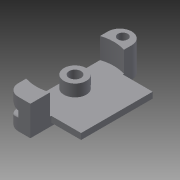
# Autodesk Inventor part: rodamiento
Saved by Autodesk Inventor 2015 SP1 (Build 190203100, 203)
## iProperties
Created: 2015-06-16
Part Number: rodamiento
Material: Generic
Document SubType Name: Modeling
Designer: pc
Density: 1 g/cm^3
Appearance: Default
Author: pc
Autodesk Inventor part; units mm, degrees
ref_plane "YZ Plane" through (0, 0, 0) normal (1, 0, 0) x (0, 1, 0)
ref_plane "XZ Plane" through (0, 0, 0) normal (0, 1, 0) x (-1, 0, 0)
ref_plane "XY Plane" through (0, 0, 0) normal (0, 0, 1) x (1, 0, 0)
sketch "Sketch1" plane through (0, 0, 0) normal (0, 0, 1) x (1, 0, 0)
  line L0 (0, -15) -> (0, 15) construction
  line L1 (-4, -15) -> (-4, 15)
  line L2 (4, 15) -> (4, -15)
  arc A0 (-4, -15) -> (0, -19) centre (0, -15) ccw
  arc A1 (4, 15) -> (-4, 15) centre (0, 15) ccw
  line L3 (4, -15) -> (0, -15)
  line L4 (-4, -11) -> (-4, -19)
  line L5 (-4, -19) -> (4, -19)
  line L6 (4, -19) -> (4, -15)
  point P0 (0, 0)
  point P1 (0, 0)
  dimension "d0" = 4
  dimension "d17" = 30
  constraints: 16 end point, 4 point on circle, 4 tangent, 3 parallel, 2 centre point, 2 midpoint, 1 coincident, 1 horizontal, 1 perpendicular, 1 point on line, 1 vertical
  measures "d0" radius of A0
  measures "d17" distance of L0.start L0.end
extrude "Extrusion1" add sketch "Sketch1" along normal blind 10 contours L1 A1 L2 L6 L5 A0
sketch "Sketch2" plane through (0, 0, 10) normal (0, 0, 1) x (1, 0, 0)
  line L0 (-4, 15) -> (-4, -15) projected
  arc A0 (-4, -15) -> (0, -19) centre (0, -15) ccw projected
  line L1 (4, -19) -> (4, 15) projected
  arc A1 (4, 15) -> (-4, 15) centre (0, 15) ccw projected
  circle A2 centre (0, 0) radius 13
  circle A3 centre (0, 0) radius 3.75
  line L2 (0, -19) -> (4, -19) projected
  dimension "d3" = 26
  dimension "d4" = 7.5
  constraints: 2 centre point, 2 coincident
  measures "d3" diameter of A2
  measures "d4" diameter of A3
extrude "Extrusion2" cut sketch "Sketch2" against normal blind 7 contours A2 L1 L0 | L0 A2 | A2 L1
sketch "Sketch3" plane through (0, 0, 10) normal (0, 0, 1) x (1, 0, 0)
  circle A0 centre (0, 0) radius 3.75 projected
  circle A1 centre (0, 0) radius 2
  line L0 (-4, 15) -> (-4, 12.3693) projected
  line L1 (4, -19) -> (4, -12.3693) projected
  arc A2 (4, 12.3693) -> (-4, 12.3693) centre (0, 0) ccw projected
  line L2 (4, 12.3693) -> (4, 15) projected
  arc A3 (4, 15) -> (-4, 15) centre (0, 15) ccw projected
  arc A4 (-4, -12.3693) -> (4, -12.3693) centre (0, 0) ccw projected
  line L3 (-4, -12.3693) -> (-4, -15) projected
  arc A5 (-4, -15) -> (0, -19) centre (0, -15) ccw projected
  line L4 (0, -19) -> (4, -19) projected
  dimension "d7" = 4
  constraints: 1 centre point, 1 coincident
  measures "d7" diameter of A1
extrude "Extrusion3" cut sketch "Sketch3" against normal through all contours A1
sketch "Sketch4" plane through (0, 0, 0) normal (0, 0, -1) x (-1, 0, 0)
  circle A0 centre (0, 0) radius 2 projected
  line L0 (4, -15) -> (4, 15) projected
  arc A1 (4, 15) -> (-4, 15) centre (0, 15) ccw projected
  line L1 (-4, 15) -> (-4, -19) projected
  arc A2 (0, -19) -> (4, -15) centre (0, -15) ccw projected
  circle A3 centre (0, 0) radius 2 projected
  line L2 (1.5898, -2.7772) -> (-1.6102, -2.7654)
  line L3 (-1.6102, -2.7654) -> (-3.2, 0.0118)
  line L4 (-3.2, 0.0118) -> (-1.5898, 2.7772)
  line L5 (-1.5898, 2.7772) -> (1.6102, 2.7654)
  line L6 (1.6102, 2.7654) -> (3.2, -0.0118)
  line L7 (3.2, -0.0118) -> (1.5898, -2.7772)
  circle A4 centre (0, 0) radius 3.2
  line L8 (-4, -19) -> (0, -19) projected
  dimension "d10" = 6.4
  constraints: 12 end point, 3 coincident, 16 other
extrude "Extrusion4" cut sketch "Sketch4" against normal blind 3 contours L2 L3 L4 L5 L6 L7
sketch "Sketch8" plane through (0, 0, 10) normal (0, 0, 1) x (1, 0, 0)
  arc A0 (4, 12.3693) -> (-4, 12.3693) centre (0, 0) ccw projected
  line L0 (4, 12.3693) -> (4, 15) projected
  arc A1 (4, 15) -> (-4, 15) centre (0, 15) ccw projected
  line L1 (-4, 15) -> (-4, 12.3693) projected
  circle A2 centre (0, 16) radius 1.65
  dimension "d28" = 3.3
  constraints: 1 centre point
  measures "d28" diameter of A2
extrude "Extrusion8" cut sketch "Sketch8" against normal through all contours A2
sketch "Sketch9" plane through (-4, -15, 0) normal (-1, 0, 0) x (0, 0, 1)
  line L0 (0, 0) -> (10, 0) projected
  line L1 (5, 0) -> (5, -2.3027) construction
  line L2 (3, 0) -> (3, -2.3027)
  line L3 (7, -2.3027) -> (7, 0)
  arc A0 (7, 0) -> (3, 0) centre (5, 0) ccw
  arc A1 (3, -2.3027) -> (7, -2.3027) centre (5, -2.3027) ccw
  line L4 (3, 2.6307) -> (3, 27.3693) projected
  point P0 (0, 15)
  point P1 (5, -1.1513)
  dimension "d31" = 4
  dimension "d34" = 2
  constraints: 8 end point, 4 point on circle, 4 tangent, 2 centre point, 2 midpoint, 1 parallel, 1 perpendicular
  measures "d31" diameter of A1
  measures "d34" distance from line of point (5, -1.151) L4
extrude "Extrusion9" cut sketch "Sketch9" against normal blind 4
sketch "Sketch10" plane through (0, 0, 10) normal (0, 0, 1) x (1, 0, 0)
  circle A0 centre (0, 0) radius 2 projected
  circle A1 centre (0, 0) radius 2 projected
  circle A2 centre (0, 0) radius 3.75 projected
extrude "Extrusion10" cut sketch "Sketch10" against normal blind 3
sketch "Sketch12" plane through (4, -19, 0) normal (1, 0, 0) x (0, 0, -1)
  line L0 (-3, 19.0118) -> (-1, 19.0118)
  line L1 (-1, 19.0118) -> (-1, 7.0118)
  line L2 (-1, 7.0118) -> (-3, 7.0118)
  line L3 (-3, 7.0118) -> (-3, 19.0118)
  line L4 (-1, 19.0118) -> (-1, 31.0118)
  line L5 (-1, 31.0118) -> (-3, 31.0118)
  line L6 (-3, 31.0118) -> (-3, 19.0118)
  point P0 (0, 19)
  dimension "d40" = 12
  dimension "d41" = 2
  constraints: 14 end point, 2 parallel, 2 symmetric about line, 1 horizontal, 1 perpendicular
  measures "d40" distance of L0.end L1.end
  measures "d41" distance of L1.end L2.end
extrude "Extrusion11" add sketch "Sketch12" along normal blind 10
body "Solid1"
